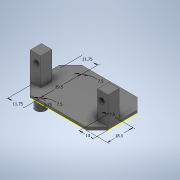
# Autodesk Inventor part: RCT-P002_servo_plate_mount
Saved by Autodesk Inventor 2020 (Build 240168000, 168)
## iProperties
Created: 2019-12-03
Part Number: RCT-P002_servo_plate_mount
Material: Generic
Document SubType Name: Modeling
Designer: maste
Density: 1 g/cm^3
Appearance: Smooth - Black
Author: maste
Autodesk Inventor part; units mm, degrees
ref_plane "YZ Plane" through (0, 0, 0) normal (1, 0, 0) x (0, 1, 0)
ref_plane "XZ Plane" through (0, 0, 0) normal (0, 1, 0) x (-1, 0, 0)
ref_plane "XY Plane" through (0, 0, 0) normal (0, 0, 1) x (1, 0, 0)
sketch "Sketch1" plane through (0, 0, 0) normal (0, 1, 0) x (-1, 0, 0)
  line L0 (56, 0) -> (0, 0) construction
  line L1 (0, 0) -> (0, -37) construction
  line L2 (0, -37) -> (56, -37) construction
  line L3 (56, -37) -> (56, 0) construction
  line L4 (56, 0) -> (48, 0) construction
  line L5 (48, 0) -> (48, -8) construction
  line L6 (48, -8) -> (56, -8) construction
  line L7 (56, -8) -> (56, 0) construction
  line L8 (56, -37) -> (48, -37) construction
  line L9 (48, -37) -> (48, -29) construction
  line L10 (48, -29) -> (56, -29) construction
  line L11 (56, -29) -> (56, -37) construction
  line L12 (0, 0) -> (8, 0) construction
  line L13 (8, 0) -> (8, -8) construction
  line L14 (8, -8) -> (0, -8) construction
  line L15 (0, -8) -> (0, 0) construction
  line L16 (0, -37) -> (8, -37) construction
  line L17 (8, -37) -> (8, -29) construction
  line L18 (8, -29) -> (0, -29) construction
  line L19 (0, -29) -> (0, -37) construction
  line L20 (48, 0) -> (56, -8)
  line L21 (56, -29) -> (48, -37)
  line L22 (8, -37) -> (0, -29)
  line L23 (8, 0) -> (0, -8)
  line L24 (56, -8) -> (56, -29)
  line L25 (48, -37) -> (8, -37)
  line L26 (0, -29) -> (0, -8)
  line L27 (8, 0) -> (48, 0)
  dimension "d0" = 56
  dimension "d1" = 37
  dimension "d2" = 8
  dimension "d3" = 8
  dimension "d4" = 8
  dimension "d5" = 8
  dimension "d6" = 8
  dimension "d7" = 8
  dimension "d8" = 8
  dimension "d9" = 8
  constraints: 56 end point, 10 parallel, 7 perpendicular, 5 horizontal, 2 collinear, 1 coincident
  measures "d0" distance of L0.start L0.end
  measures "d1" distance of L0.end L1.end
  measures "d2" distance of L6.end L5.end
  measures "d3" distance of L4.end L5.end
  measures "d4" distance of L9.end L10.end
  measures "d5" distance of L8.end L9.end
  measures "d6" distance of L12.end L13.end
  measures "d7" distance of L13.end L14.end
  measures "d8" distance of L17.end L18.end
  measures "d9" distance of L16.end L17.end
extrude "Extrusion1" add sketch "Sketch1" along normal blind 2
sketch "Sketch2" plane through (0, 2, 0) normal (0, 1, 0) x (1, 0, 0)
  line L0 (-56, 29) -> (-56, 8) projected
  line L1 (-56, 8) -> (-48.5, 8)
  line L2 (-48.5, 8) -> (-48.5, 16)
  line L3 (-48.5, 16) -> (-56, 16)
  line L4 (-56, 16) -> (-56, 8)
  line L5 (-8, 0) -> (0, 8) projected
  line L6 (0, 8) -> (-7.5, 8)
  line L7 (-7.5, 8) -> (-7.5, 16)
  line L8 (-7.5, 16) -> (0, 16)
  line L9 (0, 16) -> (0, 8)
  point P0 (0, 0)
  dimension "d12" = 8
  dimension "d13" = 7.5
  dimension "d14" = 8
  dimension "d15" = 7.5
  constraints: 16 end point, 4 parallel, 2 horizontal, 2 perpendicular
  measures "d12" distance of L1.end L2.end
  measures "d13" distance of L2.end L3.end
  measures "d14" distance of L6.end L7.end
  measures "d15" distance of L7.end L8.end
extrude "Extrusion2" add sketch "Sketch2" along normal blind 20
sketch "Sketch3" plane through (-56, 2, -8) normal (0, 0, 1) x (1, 0, 0)
  circle A0 centre (4.5, 14) radius 2
  line L0 (8, 0) -> (48, 0) projected
  line L1 (7.5, 0) -> (7.5, 20) projected
  circle A1 centre (51.5, 14) radius 2
  line L2 (48.5, 0) -> (48.5, 20) projected
  point P0 (56, -2)
  dimension "d18" = 14
  dimension "d19" = 3
  dimension "d20" = 4
  dimension "d21" = 14
  dimension "d22" = 3
  dimension "d23" = 4
  constraints: 2 centre point
  measures "d18" distance from line of L0 A0.centre
  measures "d19" distance from line of L1 A0.centre
  measures "d20" diameter of A0
  measures "d21" distance from line of L0 A1.centre
  measures "d22" distance from line of L2 A1.centre
  measures "d23" diameter of A1
extrude "Extrusion3" cut sketch "Sketch3" against normal through all
sketch "Sketch4" plane through (0, 0, 0) normal (0, -1, 0) x (1, 0, 0)
  circle A0 centre (-10, -18.5) radius 3.75
  line L0 (0, -8) -> (0, -29) projected
  line L1 (-48, 0) -> (-8, 0) projected
  circle A1 centre (-44.25, -3.75) radius 3.75
  circle A2 centre (-44.25, -33.25) radius 3.75
  line L2 (-56, -29) -> (-56, -8) projected
  point P0 (0, 0)
  dimension "d26" = 7.5
  dimension "d27" = 10
  dimension "d28" = 18.5
  dimension "d29" = 7.5
  dimension "d30" = 7.5
  dimension "d31" = 29.5
  dimension "d32" = 3.75
  dimension "d33" = 11.75
  dimension "d34" = 11.75
  constraints: 3 centre point
  measures "d26" diameter of A0
  measures "d27" distance from line of L0 A0.centre
  measures "d28" distance from line of L1 A0.centre
  measures "d29" diameter of A1
  measures "d30" diameter of A2
  measures "d31" distance of A2.centre A1.centre
  measures "d32" distance from line of L1 A1.centre
  measures "d33" distance from line of L2 A1.centre
  measures "d34" distance from line of L2 A2.centre
extrude "Extrusion4" add sketch "Sketch4" along normal blind 6 contours A1 | A2
extrude "Extrusion5" add sketch "Sketch4" along normal blind 5 contours A0
body "Solid1"
